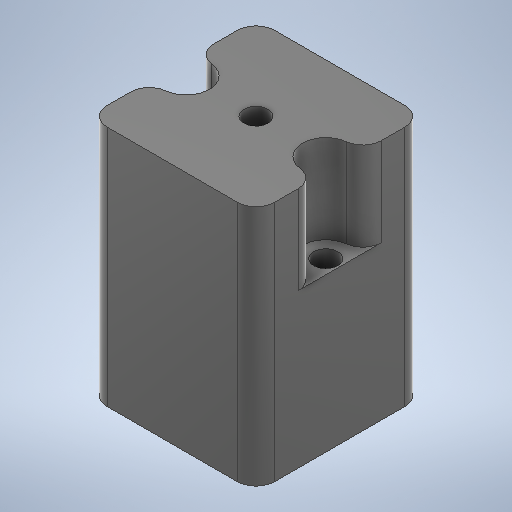
# Autodesk Inventor part: LED Power Box (12V) Pillar
Saved by Autodesk Inventor 2026.2 (Build 302298010, 298A)
## iProperties
Created: 2026-05-25
Part Number: LED Power Box (12V) Pillar
Material: ABS Plastic
Document SubType Name: Modeling
Designer: chanh
Density: 1.06 g/cm^3
Appearance: Smooth - White
Author: chanh
Autodesk Inventor part; units mm, degrees
ref_plane "YZ Plane" through (0, 0, 0) normal (1, 0, 0) x (0, 1, 0)
ref_plane "XZ Plane" through (0, 0, 0) normal (0, 1, 0) x (-1, 0, 0)
ref_plane "XY Plane" through (0, 0, 0) normal (0, 0, 1) x (1, 0, 0)
sketch "Sketch1" plane through (0, 0, 0) normal (0, 1, 0) x (-1, 0, 0)
  line L0 (18, 18) -> (-18, 18)
  line L1 (-18, 18) -> (-18, -18)
  line L2 (-18, -18) -> (18, -18)
  line L3 (18, -18) -> (18, 18)
  line L4 (18, 18) -> (-18, -18) construction
  line L5 (-18, 18) -> (18, -18) construction
  point P0 (0, 0)
  dimension "d0" = 36
  dimension "d1" = 36
  constraints: 12 end point, 2 midpoint, 2 parallel, 1 horizontal, 1 perpendicular
  measures "d0" distance of L1.end L2.end
  measures "d1" distance of L0.end L1.end
extrude "Extrusion1" add sketch "Sketch1" along normal blind 5
sketch "Sketch2" plane through (0, 5, 0) normal (0, 1, 0) x (1, 0, 0)
  line L0 (18, -18) -> (18, 18) projected
  line L1 (18, 18) -> (-18, 18) projected
  line L2 (-18, 18) -> (-18, -18) projected
  line L3 (-18, -18) -> (18, -18) projected
  line L4 (-18, -18) -> (18, -18)
  line L5 (18, -18) -> (18, 18)
  line L6 (18, 18) -> (-18, 18)
  line L7 (-18, 18) -> (-18, -18)
  line L8 (-18, -18) -> (18, 18) construction
  line L9 (18, -18) -> (-18, 18) construction
  point P0 (0, 0)
  constraints: 12 end point, 2 midpoint, 2 parallel, 2 perpendicular, 1 horizontal, 1 point on line
extrude "Extrusion2" add sketch "Sketch2" along normal blind 47
sketch "Sketch3" plane through (0, 52, 0) normal (0, 1, 0) x (1, 0, 0)
  line L0 (-15, 0) -> (15, 0) construction
  point P0 (0, 0)
  point P1 (0, 0)
  dimension "d6" = 30
  constraints: 3 coincident, 2 end point, 1 horizontal, 1 midpoint
  measures "d6" distance of L0.start L0.end
hole "Hole1" at (-15, 52, 0) at (15, 52, 0) direction (0, -1, 0) diameter 5.2 end through all counterbore diameter 10 counterbore depth 19
fillet "Fillet1" radius 4 8 edges at (18, 26, 18) (-18, 26, 18) (18, 26, -18) (-18, 26, -18) (18, 42.5, -4) (18, 42.5, 4) (-18, 42.5, 4) (-18, 42.5, -4)
sketch "Sketch4" plane through (0, 52, 0) normal (0, 1, 0) x (1, 0, 0)
  point P0 (0, 0)
  point P1 (0, 0)
  constraints: 1 coincident
hole "Hole2" at (0, 52, 0) direction (0, -1, 0) diameter 5.2 depth 20
body "Solid1"
